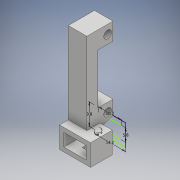
# Autodesk Inventor part: Proximity Sensor Mount_1
Saved by Autodesk Inventor 2017 (Build 210142000, 142)
## iProperties
Created: 2017-05-01
Part Number: Proximity Sensor Mount_1
Material: Generic
Document SubType Name: Modeling
Designer: willt
Density: 1 g/cm^3
Appearance: Default
Author: willt
Autodesk Inventor part; units mm, degrees
ref_plane "YZ Plane" through (0, 0, 0) normal (1, 0, 0) x (0, 1, 0)
ref_plane "XZ Plane" through (0, 0, 0) normal (0, 1, 0) x (-1, 0, 0)
ref_plane "XY Plane" through (0, 0, 0) normal (0, 0, 1) x (1, 0, 0)
sketch "Sketch1" plane through (0, 0, 0) normal (1, 0, 0) x (0, 1, 0)
  line L0 (0, 0) -> (0, -8)
  line L1 (0, -8) -> (-7, -8)
  line L2 (-7, -8) -> (-7, -31)
  line L3 (-7, -31) -> (0, -31)
  line L4 (0, -31) -> (0, -37.5)
  line L5 (0, -37.5) -> (-12, -37.5)
  line L6 (-12, -37.5) -> (-12, 0)
  line L7 (-12, 0) -> (0, 0)
  line L8 (0, -4) -> (-2.5, -4) construction
  circle A0 centre (-2.5, -4) radius 1.75
  line L9 (0, -31) -> (-2.5, -31) construction
  line L10 (-2.5, -31) -> (-2.5, -35) construction
  circle A1 centre (-2.5, -35) radius 1.75
  dimension "d0" = 8
  dimension "d1" = 7
  dimension "d2" = 23
  dimension "d3" = 6.5
  dimension "d4" = 12
  dimension "d5" = 2.5
  dimension "d6" = 3.5
  dimension "d7" = 4
  dimension "d8" = 3.5
  constraints: 22 end point, 7 perpendicular, 3 point on line, 2 centre point, 2 coincident, 1 horizontal, 1 midpoint, 1 vertical
  measures "d0" distance of L0.start L0.end
  measures "d1" distance of L0.end L1.end
  measures "d2" distance of L1.end L2.end
  measures "d3" distance of L3.end L4.end
  measures "d4" distance of L4.end L5.end
  measures "d5" distance of L8.start L8.end
  measures "d6" diameter of A0
  measures "d7" distance of L9.end L10.end
  measures "d8" diameter of A1
extrude "Extrusion1" add sketch "Sketch1" along normal blind 8.5
sketch "Sketch2" plane through (0, 0, -31) normal (0, 1, 0) x (1, 0, 0)
  line L0 (0, 6.5) -> (0, -31) projected
  line L1 (0, 6.5) -> (2, 6.5) construction
  line L2 (0, 6.5) -> (8.5, 6.5) construction
  line L3 (2, 6.5) -> (0, 6.5) construction
  line L4 (0, 16.3) -> (2, 16.3) construction
  line L5 (2, 16.3) -> (2, 14.3) construction
  line L6 (2, 14.3) -> (12.2, 14.3)
  line L7 (12.2, 14.3) -> (12.2, 8.5)
  line L8 (12.2, 8.5) -> (2, 8.5)
  line L9 (2, 8.5) -> (2, 14.3)
  line L10 (0, 6.5) -> (14.2, 6.5)
  line L11 (14.2, 6.5) -> (14.2, 16.3)
  line L12 (14.2, 16.3) -> (0, 16.3)
  line L13 (0, 16.3) -> (0, 6.5)
  dimension "d11" = 9.8
  dimension "d15" = 2
  dimension "d16" = 2
  dimension "d17" = 10.2
  dimension "d18" = 5.8
  dimension "d19" = 14.2
  constraints: 24 end point, 4 parallel, 3 perpendicular, 2 horizontal, 1 collinear, 1 point on line
  measures "d11" distance of point (0, 6.5) L4.start
  measures "d15" distance of L4.start L4.end
  measures "d16" distance of L4.end L5.end
  measures "d17" distance of L7.end L8.end
  measures "d18" distance of L6.end L7.end
  measures "d19" distance of L12.end L11.end
extrude "Extrusion2" add sketch "Sketch2" against normal blind 16
extrude "Extrusion3" cut sketch "Sketch2" against normal blind 6
sketch "Sketch3" plane through (8.5, 0, 0) normal (1, 0, 0) x (0, 0, -1)
  line L0 (37.5, 0) -> (31, 0) projected
  line L1 (37.5, 0) -> (39.5451, -6)
  line L2 (37.5, -12) -> (37.5, -6) projected
  line L3 (39.5451, -6) -> (37.5, -6)
  line L4 (37.5, -6) -> (37.5, 0)
  point P0 (0, 0)
  constraints: 6 end point, 2 perpendicular
extrude "Extrusion4" add sketch "Sketch3" against normal blind 8.5
sketch "Sketch4" plane through (2, -16, -45.3) normal (0, 0, 1) x (1, 0, 0)
  line L0 (10.2, 0) -> (0, 0) construction
  line L1 (5.1, 0) -> (5.1, 4) construction
  line L2 (10.2, 10) -> (0, 10) construction
  line L3 (5.1, 4) -> (4.35, 4) construction
  line L4 (4.35, 4) -> (5.85, 4)
  line L5 (5.85, 4) -> (5.85, 6)
  line L6 (5.85, 6) -> (4.35, 6)
  line L7 (4.35, 6) -> (4.35, 4)
  point P0 (-2, 16)
  dimension "d28" = 1.5
  dimension "d29" = 2
  constraints: 12 end point, 3 perpendicular, 2 parallel, 1 horizontal, 1 midpoint
  measures "d28" distance of L6.end L5.end
  measures "d29" distance of L5.end L4.end
extrude "Extrusion5" cut sketch "Sketch4" against normal blind 1
sketch "Sketch5" plane through (12.2, -16, -39.5) normal (0, 0, -1) x (-1, 0, 0)
  line L0 (10.2, 0) -> (0, 0) construction
  line L1 (5.1, 0) -> (5.1, 4) construction
  line L2 (5.1, 4) -> (4.35, 4) construction
  line L3 (4.35, 4) -> (5.85, 4)
  line L4 (5.85, 4) -> (5.85, 6)
  line L5 (5.85, 6) -> (4.35, 6)
  line L6 (4.35, 6) -> (4.35, 4)
  point P0 (12.2, 16)
  dimension "d34" = 1.5
  dimension "d35" = 2
  constraints: 12 end point, 2 parallel, 2 perpendicular, 1 horizontal, 1 midpoint, 1 vertical
  measures "d34" distance of L5.end L4.end
  measures "d35" distance of L4.end L3.end
extrude "Extrusion6" cut sketch "Sketch5" against normal blind 1
body "Solid1"
